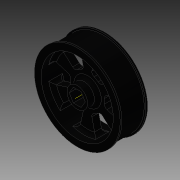
# Autodesk Inventor part: Wheel V1
Saved by Autodesk Inventor 2013 (Build 170138000, 138)
## iProperties
Created: 2013-04-01
Part Number: Wheel V1
Material: Generic
Document SubType Name: Modeling
Designer: mvarma
Density: 1 g/cm^3
Author: mvarma
Autodesk Inventor part; units mm, degrees
ref_plane "YZ Plane" through (0, 0, 0) normal (1, 0, 0) x (0, 1, 0)
ref_plane "XZ Plane" through (0, 0, 0) normal (0, 1, 0) x (-1, 0, 0)
ref_plane "XY Plane" through (0, 0, 0) normal (0, 0, 1) x (1, 0, 0)
sketch "Sketch1" plane through (0, 0, 0) normal (0, 0, 1) x (1, 0, 0)
  circle A0 centre (0, 0) radius 9.525
  circle A1 centre (0, 0) radius 15.875
  circle A2 centre (0, 0) radius 38.1
  circle A3 centre (0, 0) radius 33.3375
  line L0 (-7.3323, 0) -> (-3.6662, 6.35)
  line L1 (-3.6662, 6.35) -> (3.6662, 6.35)
  line L2 (3.6662, 6.35) -> (7.3323, 0)
  line L3 (7.3323, 0) -> (3.6662, -6.35)
  line L4 (3.6662, -6.35) -> (-3.6662, -6.35)
  line L5 (-3.6662, -6.35) -> (-7.3323, 0)
  line L6 (0, 0) -> (-8.2463, 37.1969)
  line L7 (0, 0) -> (8.2463, 37.1969)
  line L8 (0, 38.1) -> (0, 0)
  line L9 (0, 0) -> (-36.3366, 11.4569)
  line L10 (0, 0) -> (-28.0903, 25.74)
  line L11 (0, 0) -> (-28.0903, -25.74)
  line L12 (0, 0) -> (-36.3366, -11.4569)
  line L13 (0, 0) -> (8.2463, -37.1969)
  line L14 (0, 0) -> (-8.2463, -37.1969)
  line L15 (0, 0) -> (36.3366, -11.4569)
  line L16 (0, 0) -> (28.0903, -25.74)
  line L17 (0, 0) -> (28.0903, 25.74)
  line L18 (0, 0) -> (36.3366, 11.4569)
  dimension "d0" = 76.2
  dimension "d2" = 66.675
  dimension "d3" = 19.05
  dimension "d4" = 31.75
  dimension "d5" = 12.7
  dimension "d6" = 12.5
  dimension "d7" = 12.5
  dimension "d10" = 360
  constraints: 38 end point, 5 coincident, 4 centre point, 3 point on circle, 1 horizontal, 1 perpendicular, 44 other
  measures "d0" diameter of A2
  measures "d2" diameter of A3
  measures "d3" diameter of A0
  measures "d4" diameter of A1
  measures "d5" distance between parallel lines of L4 L1
  measures "d6" angle of L6 L8
  measures "d7" angle of L8 L7
extrude "Extrusion1" add sketch "Sketch1" along normal blind 12.7 contours A0 L15 L3 L2 L18 | L18 L2 L17 A0 | A0 L16 L3 L15 | L17 L2 L1 L7 A0 | L18 L17 L2 | L2 L3 L15 L18 | A0 L13 L4 L3 L16 | L3 L16 L15 | L7 L1 L8 A0 | L17 L7 L1 L2 | L10 L0 L1 L6 | L8 L1 L7 | L6 L1 L8 | L12 L5 L0 L9 | L9 L0 L10 | L14 L4 L5 L11 | L11 L5 L12 | L16 L3 L4 L13 | L13 L4 L14 | A0 L14 L4 L13 | L8 L1 L6 A0 | L1 L0 L10 A0 L6 | L9 A0 L10 L0 | L0 L5 L12 A0 L9 | L11 A0 L12 L5 | L5 L4 L14 A0 L11
extrude "Extrusion2" add sketch "Sketch1" along normal blind 3.175 contours A0 L18 A1 L15 | A0 L17 A1 L18 | L15 A1 L16 A0 | A0 L7 A1 L17 | L16 A1 L13 A0 | A0 L8 A1 L7 | L13 A1 L14 A0 | A0 L6 A1 L8 | L14 A1 L11 A0 | A0 L10 A1 L6 | L9 A1 L10 A0 | A0 L12 A1 L9 | L11 A1 L12 A0
extrude "Extrusion3" add sketch "Sketch1" along normal blind 12.7 contours L18 A2 L15 A3 | A3 L17 A2 L18 | L15 A2 L16 A3 | A3 L7 A2 L17 | L16 A2 L13 A3 | A3 L8 A2 L7 | L13 A2 L14 A3 | A3 L6 A2 L8 | L14 A2 L11 A3 | A3 L10 A2 L6 | L9 A2 L10 A3 | A3 L12 A2 L9 | L11 A2 L12 A3
extrude "Extrusion4" add sketch "Sketch1" along normal up to surface (3.175 mm away) contours L18 L17 L2 | L2 L3 L15 L18 | L3 L16 L15 | L7 L1 L8 A0 | A0 L8 A1 L7 | L17 L7 L1 L2 | L10 L0 L1 L6 | L8 L1 L7 | L6 L1 L8 | L12 L5 L0 L9 | L9 L0 L10 | L14 L4 L5 L11 | L11 L5 L12 | L16 L3 L4 L13 | L13 L4 L14 | L8 L1 L6 A0 | A0 L6 A1 L8 | A1 L8 A3 L7 | A1 L6 A3 L8 | A3 L8 A2 L7 | A3 L6 A2 L8
pattern_circular "Circular Pattern1" count 6 over 360 about axis through (0, 0, 0) along (0, 0, -1) of "Extrusion4"
fillet "Fillet1" radius 3.175 4 edges at (7.2156, 32.5473, 1.5875) (3.436, 15.4987, 1.5875) (24.579, 22.5225, 1.5875) (11.7043, 10.725, 1.5875)
pattern_circular "Circular Pattern2" count 6 over 360 about axis through (0, 0, 0) along (0, 0, -1) of "Fillet1"
fillet "Fillet2" radius 3.175 19 edges at (-8.9209, 32.1217, 3.175) (0, 33.3375, 3.175) (8.9209, 32.1217, 3.175) (23.3578, 23.7866, 3.175) (28.8711, 16.6688, 3.175) (32.2787, 8.3351, 3.175) (32.2787, -8.3351, 3.175) (28.8711, -16.6687, 3.175) (23.3578, -23.7866, 3.175) (-8.9209, -32.1217, 3.175) (0, -33.3375, 3.175) (8.9209, -32.1217, 3.175) (-32.2787, -8.3351, 3.175) (-28.8711, -16.6688, 3.175) (-23.3578, -23.7866, 3.175) (-23.3578, 23.7866, 3.175) (-28.8711, 16.6687, 3.175) (-32.2787, 8.3351, 3.175) (-9.525, 0, 3.175)
extrude "Extrusion5" cut sketch "Sketch1" along normal up to next contours L18 L17 L2 | L2 L3 L15 L18 | L3 L16 L15 | L17 L7 L1 L2 | L10 L0 L1 L6 | L8 L1 L7 | L6 L1 L8 | L12 L5 L0 L9 | L9 L0 L10 | L14 L4 L5 L11 | L11 L5 L12 | L16 L3 L4 L13 | L13 L4 L14
sketch "Sketch2" plane through (0, 0, 12.7) normal (0, 0, 1) x (1, 0, 0)
  circle A0 centre (0, 0) radius 38.1 projected
  circle A1 centre (0, 0) radius 39.6875
  dimension "d30" = 79.375
  constraints: 1 centre point, 1 coincident
  measures "d30" diameter of A1
extrude "Extrusion6" add sketch "Sketch2" against normal blind 1.5875
mirror "Mirror1" about plane through (0, 0, 0) normal (0, 0, -1)
equation "\"d6\" = d7"
body "Solid1"
